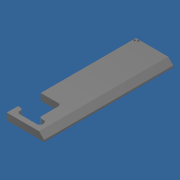
# Autodesk Inventor part: Front_Cover
Saved by Autodesk Inventor 2020 (Build 240168000, 168)
## iProperties
Created: 2021-05-18
Part Number: Front_Cover
Material: 一般
Document SubType Name: Modeling
Designer: ken113
Density: 1 g/cm^3
Appearance: 滑らか - 黒
Author: ken113
Autodesk Inventor part; units mm, degrees
ref_plane "YZ Plane" through (0, 0, 0) normal (1, 0, 0) x (0, 1, 0)
ref_plane "XZ Plane" through (0, 0, 0) normal (0, 1, 0) x (-1, 0, 0)
ref_plane "XY Plane" through (0, 0, 0) normal (0, 0, 1) x (1, 0, 0)
sketch "スケッチ1" plane through (0, 0, 0) normal (0, 1, 0) x (-1, 0, 0)
  line L0 (-55, -190) -> (55, -190)
  line L1 (55, -190) -> (55, 190)
  line L2 (55, 190) -> (-55, 190)
  line L3 (-55, 190) -> (-55, -190)
  line L4 (-55, -190) -> (55, 190) construction
  line L5 (55, -190) -> (-55, 190) construction
  point P0 (0, 0)
  dimension "d0" = 380
  dimension "d1" = 110
  constraints: 12 end point, 2 midpoint, 2 parallel, 1 horizontal, 1 perpendicular
  measures "d0" distance of L2.end L0.start
  measures "d1" distance of L1.end L2.end
extrude "押し出し1" add sketch "スケッチ1" along normal blind 20
chamfer "面取り1" distance 15 angle 45 1 edges at (55, 20, 0)
sketch "スケッチ2" plane through (0, 20, 0) normal (0, 1, 0) x (1, 0, 0)
  line L0 (27.0676, -175) -> (-55, -175)
  line L1 (-55, -175) -> (-55, -155)
  line L2 (-55, -155) -> (27.0676, -155)
  line L3 (27.0676, -155) -> (27.0676, -175)
  line L4 (-55, -190) -> (40, -190) projected
  line L5 (-55, 190) -> (-55, -190) projected
  point P0 (0, 0)
  point P1 (-6.584, -148.8716)
  point P2 (37.9289, -190)
  dimension "d10" = 15
  dimension "d11" = 0
  dimension "d16" = 20
  constraints: 8 end point, 2 parallel, 1 horizontal, 1 perpendicular
  measures "d10" distance between parallel lines of L0 L4
  measures "d11" distance between parallel lines of L5 L1
  measures "d16" distance of L2.end L0.start
extrude "押し出し2" cut sketch "スケッチ2" against normal blind 20
sketch "スケッチ3" plane through (0, 0, 0) normal (0, -1, 0) x (1, 0, 0)
  line L0 (-55, 155) -> (5, 155)
  line L1 (5, 155) -> (5, 90)
  line L2 (5, 90) -> (-55, 90)
  line L3 (-55, 90) -> (-55, 155)
  line L4 (-55, 175) -> (27.0676, 175) projected
  point P0 (0, 0)
  dimension "d12" = 85
  dimension "d13" = 60
  constraints: 8 end point, 2 parallel, 1 horizontal, 1 perpendicular
  measures "d12" distance between parallel lines of L2 L4
  measures "d13" distance of L1.end L2.end
extrude "押し出し3" cut sketch "スケッチ3" against normal blind 20
sketch "スケッチ4" plane through (0, 20, 0) normal (0, 1, 0) x (1, 0, 0)
  line L0 (-55, -90) -> (5, -90) projected
  line L1 (5, -90) -> (5, -155) projected
  line L2 (5, -155) -> (27.0676, -155) projected
  line L3 (27.0676, -155) -> (27.0676, -175) projected
  line L4 (27.0676, -175) -> (-55, -175) projected
  line L5 (-55, -175) -> (-55, -190) projected
  line L6 (-55, -190) -> (40, -190) projected
  line L7 (40, 190) -> (-55, 190) projected
  line L8 (-55, 190) -> (-55, -90) projected
  line L9 (-55, -175) -> (-55, -190) projected
  line L10 (-55, -175) -> (-40, -175)
  line L11 (-40, -175) -> (-40, -157)
  line L12 (-40, -157) -> (-55, -157)
  line L13 (-55, -157) -> (-55, -175)
  line L14 (40, 190) -> (40, -190) projected
  point P0 (0, 0)
  dimension "d17" = 18
  dimension "d18" = 15
  constraints: 8 end point, 2 parallel, 1 horizontal, 1 perpendicular
  measures "d17" distance of L10.end L11.end
  measures "d18" distance of L11.end L12.end
extrude "押し出し4" add sketch "スケッチ4" against normal blind 20 contours L4 L13 L12 L11
chamfer "面取り2" distance 5 angle 45 6 edges at (5, 10, 90) (5, 10, 155) (27.0676, 10, 155) (27.0676, 10, 175) (-40, 10, 175) (-40, 10, 157)
fillet "フィレット2" radius 2 12 edges at (-45, 10, 157) (-40, 10, 162) (-40, 10, 170) (-35, 10, 175) (22.0676, 10, 175) (27.0676, 10, 170) (27.0676, 10, 160) (22.0676, 10, 155) (10, 10, 155) (5, 10, 150) (5, 10, 95) (0, 10, 90)
shell "シェル1" thickness 4 removed faces 1 at (-0.2761, 0, -96.6667)
sketch "スケッチ14" plane through (0, 20, 0) normal (0, 1, 0) x (1, 0, 0)
  arc A0 (21.2391, -179) -> (25.4818, -177.2426) centre (21.2391, -173) ccw projected
  line L0 (21.2391, -179) -> (-34.1716, -179) projected
  arc A1 (-38.4142, -177.2426) -> (-34.1716, -179) centre (-34.1716, -173) ccw projected
  line L1 (-38.4142, -177.2426) -> (-42.2426, -173.4142) projected
  arc A2 (-44, -169.1716) -> (-42.2426, -173.4142) centre (-38, -169.1716) ccw projected
  line L2 (-44, -169.1716) -> (-44, -163.6569) projected
  line L3 (-44, -163.6569) -> (-46.6569, -161) projected
  line L4 (-46.6569, -161) -> (-51, -161) projected
  line L5 (-51, -161) -> (-51, -186) projected
  line L6 (-51, -186) -> (51, -186) projected
  line L7 (51, -186) -> (51, 186) projected
  line L8 (51, 186) -> (-51, 186) projected
  line L9 (-51, 186) -> (-51, -86) projected
  line L10 (-51, -86) -> (-0.8284, -86) projected
  arc A3 (3.4142, -87.7574) -> (-0.8284, -86) centre (-0.8284, -92) ccw projected
  line L11 (3.4142, -87.7574) -> (7.2426, -91.5858) projected
  arc A4 (9, -95.8284) -> (7.2426, -91.5858) centre (3, -95.8284) ccw projected
  line L12 (9, -95.8284) -> (9, -148.3431) projected
  line L13 (9, -148.3431) -> (11.6569, -151) projected
  line L14 (11.6569, -151) -> (21.2391, -151) projected
  arc A5 (25.4818, -152.7574) -> (21.2391, -151) centre (21.2391, -157) ccw projected
  line L15 (25.4818, -152.7574) -> (29.3102, -156.5858) projected
  arc A6 (31.0676, -160.8284) -> (29.3102, -156.5858) centre (25.0676, -160.8284) ccw projected
  line L16 (31.0676, -160.8284) -> (31.0676, -169.1716) projected
  arc A7 (29.3102, -173.4142) -> (31.0676, -169.1716) centre (25.0676, -169.1716) ccw projected
  line L17 (29.3102, -173.4142) -> (25.4818, -177.2426) projected
  arc A8 (5, -149.1716) -> (5.5858, -150.5858) centre (7, -149.1716) ccw projected
  line L18 (5, -149.1716) -> (5, -95.8284) projected
  arc A9 (5, -95.8284) -> (4.4142, -94.4142) centre (3, -95.8284) ccw projected
  line L19 (0.5858, -90.5858) -> (4.4142, -94.4142) projected
  arc A10 (0.5858, -90.5858) -> (-0.8284, -90) centre (-0.8284, -92) ccw projected
  line L20 (-0.8284, -90) -> (-55, -90) projected
  line L21 (-55, 190) -> (-55, -90) projected
  line L22 (55, 190) -> (-55, 190) projected
  line L23 (55, -190) -> (55, 190) projected
  line L24 (-55, -190) -> (55, -190) projected
  line L25 (-55, -157) -> (-55, -190) projected
  line L26 (-55, -157) -> (-45.8284, -157) projected
  arc A11 (-44.4142, -157.5858) -> (-45.8284, -157) centre (-45.8284, -159) ccw projected
  line L27 (-40.5858, -161.4142) -> (-44.4142, -157.5858) projected
  arc A12 (-40, -162.8284) -> (-40.5858, -161.4142) centre (-42, -162.8284) ccw projected
  line L28 (-40, -162.8284) -> (-40, -169.1716) projected
  arc A13 (-40, -169.1716) -> (-39.4142, -170.5858) centre (-38, -169.1716) ccw projected
  line L29 (-35.5858, -174.4142) -> (-39.4142, -170.5858) projected
  arc A14 (-35.5858, -174.4142) -> (-34.1716, -175) centre (-34.1716, -173) ccw projected
  line L30 (-34.1716, -175) -> (21.2391, -175) projected
  arc A15 (21.2391, -175) -> (22.6534, -174.4142) centre (21.2391, -173) ccw projected
  line L31 (26.4818, -170.5858) -> (22.6534, -174.4142) projected
  arc A16 (26.4818, -170.5858) -> (27.0676, -169.1716) centre (25.0676, -169.1716) ccw projected
  line L32 (27.0676, -169.1716) -> (27.0676, -160.8284) projected
  arc A17 (27.0676, -160.8284) -> (26.4818, -159.4142) centre (25.0676, -160.8284) ccw projected
  line L33 (22.6534, -155.5858) -> (26.4818, -159.4142) projected
  arc A18 (22.6534, -155.5858) -> (21.2391, -155) centre (21.2391, -157) ccw projected
  line L34 (21.2391, -155) -> (10.8284, -155) projected
  arc A19 (9.4142, -154.4142) -> (10.8284, -155) centre (10.8284, -153) ccw projected
  line L35 (5.5858, -150.5858) -> (9.4142, -154.4142) projected
  line L36 (-47.5359, 186) -> (-45.8038, 189)
  line L37 (-45.8038, 189) -> (-42.3397, 189)
  line L38 (-42.3397, 189) -> (-40.6077, 186)
  line L39 (-40.6077, 186) -> (-42.3397, 183)
  line L40 (-42.3397, 183) -> (-45.8038, 183)
  line L41 (-45.8038, 183) -> (-47.5359, 186)
  line L42 (-47.5359, 182) -> (-49.2679, 179)
  line L43 (-49.2679, 179) -> (-52.7321, 179)
  line L44 (-52.7321, 179) -> (-54.4641, 182)
  line L45 (-54.4641, 182) -> (-52.7321, 185)
  line L46 (-52.7321, 185) -> (-49.2679, 185)
  line L47 (-49.2679, 185) -> (-47.5359, 182)
  point P0 (0, 0)
  point P1 (-44.0718, 186)
  point P2 (-51, 182)
  dimension "d79" = 6
  dimension "d80" = 6
  dimension "d82" = 2
  dimension "d83" = 1
  dimension "d84" = 6.9282
  dimension "d85" = 4
  constraints: 24 end point, 2 point on line, 2 vertical alignment, 1 parallel, 26 other
  measures "d79" distance between parallel lines of L37 L40
  measures "d80" distance between parallel lines of L46 L43
  measures "d82" distance between parallel lines of L41 L47
  measures "d83" distance from line of L36.start L46
  measures "d84" horizontal distance of point (-51, 182) point (-44.072, 186)
  measures "d85" vertical distance of point (-44.072, 186) point (-51, 182)
extrude "押し出し10" cut sketch "スケッチ14" against normal through all contours L39 L40 L41 L8 | L8 L36 L37 L38 | L46 L47 L42 L43 L9 | L9 L43 L44 L45 L46
